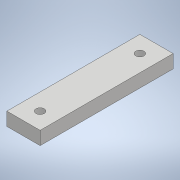
# Autodesk Inventor part: モータースペーサ
Saved by Autodesk Inventor 2022 (Build 260153000, 153)
## iProperties
Part Number: モータースペーサ
Material: 一般
Document SubType Name: Modeling
Designer: highs
Density: 1 g/cm^3
Appearance: 既定
Author: highs
## iProperties of the stored document モータースペーサ2_3D プリント.ipt
Created: 2021-07-21
Part Number: モータースペーサ2_3D プリント
Material: 一般
Document SubType Name: Modeling
Designer: chpkk
Density: 1 g/cm^3
Appearance: 既定
Author: chpkk
Autodesk Inventor part; units mm, degrees
ref_plane "YZ Plane" through (0, 0, 0) normal (1, 0, 0) x (0, 1, 0)
ref_plane "XZ Plane" through (0, 0, 0) normal (0, 1, 0) x (-1, 0, 0)
ref_plane "XY Plane" through (0, 0, 0) normal (0, 0, 1) x (1, 0, 0)
sketch "スケッチ2" plane through (0, 0, 0) normal (0, 0, 1) x (1, 0, 0)
  line L0 (0, 0) -> (20, 0)
  line L1 (20, 0) -> (20, 80)
  line L2 (20, 80) -> (0, 80)
  line L3 (0, 80) -> (0, 0)
  line L4 (10, 80) -> (10, 0) construction
  circle A0 centre (10, 70) radius 2.5
  circle A1 centre (10, 10) radius 2.5
  dimension "d4" = 20
  dimension "d5" = 80
  dimension "d15" = 10
  dimension "d16" = 10
  dimension "d17" = 5
  constraints: 10 end point, 2 centre point, 2 horizontal, 2 midpoint, 2 perpendicular, 2 point on line, 1 equal radius
  measures "d4" distance of L0.start L0.end
  measures "d5" distance of L2.end L0.start
  measures "d15" distance from line of L2 A0.centre
  measures "d16" distance from line of L0 A1.centre
  measures "d17" diameter of A0
extrude "押し出し2" add sketch "スケッチ2" along normal blind 8
